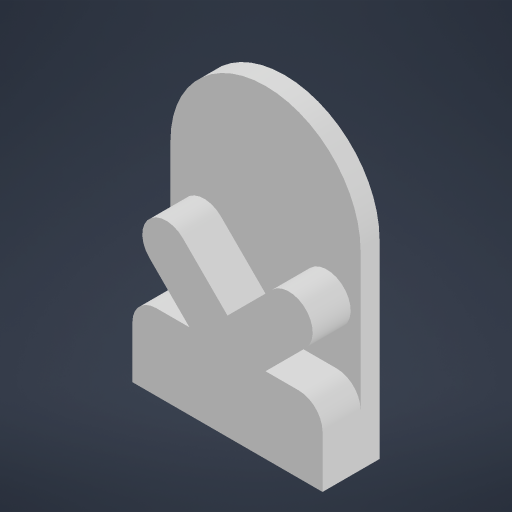
# Autodesk Inventor part: Marker Holder 90 deg
Saved by Autodesk Inventor 2024.1 (Build 281209000, 209)
## iProperties
Created: 2023-09-09
Part Number: Marker Holder 90 deg
Material: Generic
Document SubType Name: Modeling
Designer: User
Density: 1 g/cm^3
Appearance: Default
Author: User
Autodesk Inventor part; units mm, degrees
ref_plane "YZ Plane" through (0, 0, 0) normal (1, 0, 0) x (0, 1, 0)
ref_plane "XZ Plane" through (0, 0, 0) normal (0, 1, 0) x (-1, 0, 0)
ref_plane "XY Plane" through (0, 0, 0) normal (0, 0, 1) x (1, 0, 0)
sketch "Sketch9" plane through (0, 0, 0) normal (0, 0, 1) x (1, 0, 0)
  line L0 (0, 0) -> (100, 0)
  line L1 (100, 0) -> (100, 150)
  line L2 (100, 150) -> (0, 150)
  line L3 (0, 150) -> (0, 0)
  dimension "d68" = 100
  dimension "d69" = 150
  constraints: 8 end point, 2 parallel, 1 horizontal, 1 perpendicular
  measures "d68" distance of L2.end L1.end
  measures "d69" distance of L1.end L0.end
extrude "Extrusion8" add sketch "Sketch9" along normal blind 10
sketch "Sketch10" plane through (0, 0, 10) normal (0, 0, 1) x (1, 0, 0)
  line L0 (0, 150) -> (0, 0) projected
  line L1 (0, 0) -> (100, 0)
  line L2 (100, 0) -> (100, 20)
  line L3 (100, 20) -> (0, 20)
  line L4 (0, 20) -> (0, 0)
  line L5 (50, 20) -> (0, 70)
  line L6 (0, 70) -> (17.6777, 87.6777)
  line L7 (17.6777, 87.6777) -> (67.6777, 37.6777)
  line L8 (67.6777, 37.6777) -> (50, 20)
  line L9 (50, 20) -> (120.7107, 20) construction
  line L10 (50, 20) -> (100, 70)
  line L11 (100, 70) -> (82.3223, 87.6777)
  line L12 (82.3223, 87.6777) -> (32.3223, 37.6777)
  line L13 (32.3223, 37.6777) -> (50, 20)
  line L14 (50, 20) -> (120.7107, 20) construction
  line L15 (0, 20) -> (100, 20)
  line L16 (100, 20) -> (100, 40)
  line L17 (100, 40) -> (0, 40)
  line L18 (0, 40) -> (0, 20)
  point P0 (70, 40)
  point P1 (65.3553, 40)
  point P2 (50, 55.3553)
  point P3 (30, 40)
  dimension "d72" = 100
  dimension "d73" = 20
  dimension "d74" = 135
  dimension "d75" = 25
  dimension "d76" = 45
  dimension "d77" = 25
  dimension "d78" = 20
  constraints: 36 end point, 8 parallel, 4 perpendicular, 3 horizontal, 2 equal length, 1 collinear, 1 midpoint, 1 point on line
  measures "d72" distance of L3.end L2.end
  measures "d73" distance of L2.end L1.end
  measures "d74" angle of L9 L5
  measures "d75" distance of L5.end L6.end
  measures "d76" angle of L14 L10
  measures "d77" distance of L11.end L10.end
  measures "d78" distance of L16.end L2.end
extrude "Extrusion9" add sketch "Sketch10" along normal blind 20 contours L6 L7 L12 L17 L5 | L17 L5 L3 L0 | L17 L12 L5 | L3 L2 L1 L0 | L12 L17 L7 L8 L5 | L12 L7 L17 | L12 L11 L10 L17 L7 | L8 L10 L17 L16 L3 | L17 L10 L7
fillet "Fillet8" radius 50 2 edges at (0, 150, 5) (100, 150, 5)
fillet "Fillet9" radius 12.5 6 edges at (17.6777, 87.6777, 20) (0, 70, 20) (82.3223, 87.6777, 20) (100, 70, 20) (0, 40, 20) (100, 40, 20)
body "Solid3"
